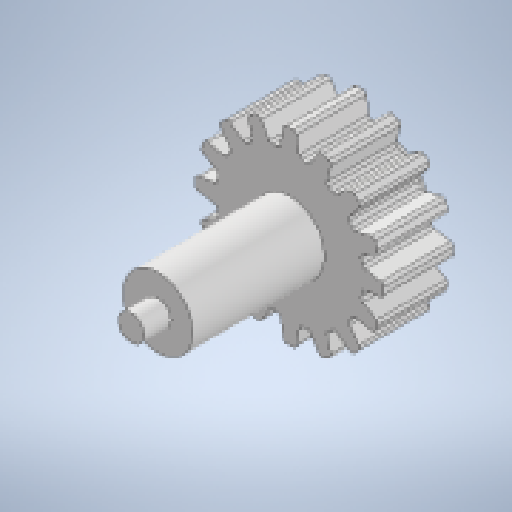
# Autodesk Inventor part: GearDirect
Saved by Autodesk Inventor 2025.2 (Build 292293000, 293)
## iProperties
Created: 2026-02-21
Part Number: GearDirect
Material: 一般
Document SubType Name: Modeling
Designer: naka6
Density: 1 g/cm^3
Appearance: 既定
Author: naka6
Autodesk Inventor part; units mm, degrees
ref_plane "YZ Plane" through (0, 0, 0) normal (1, 0, 0) x (0, 1, 0)
ref_plane "XZ Plane" through (0, 0, 0) normal (0, 1, 0) x (-1, 0, 0)
ref_plane "XY Plane" through (0, 0, 0) normal (0, 0, 1) x (1, 0, 0)
sketch "スケッチ1" plane through (0, 0, 0) normal (0, 0, 1) x (1, 0, 0)
  circle A0 centre (0, 0) radius 7 projected
  point P0 (0, 0)
extrude "押し出し1" add sketch "スケッチ1" along normal blind 3
sketch "スケッチ2" plane through (0, 0, 3) normal (0, 0, 1) x (1, 0, 0)
  circle A0 centre (0, 0) radius 13.5
  dimension "d2" = 27
  constraints: 1 centre point, 1 coincident
  measures "d2" diameter of A0
extrude "押し出し2" add sketch "スケッチ2" along normal blind 10
sketch "スケッチ3" plane through (0, 0, 13) normal (0, 0, 1) x (1, 0, 0)
  line L0 (0, 0) -> (13.5, 0)
  circle A0 centre (0, 0) radius 13.5 projected
  line L1 (0, 0) -> (13.4711, 0.8829)
  line L2 (0, 0) -> (13.3845, 1.7621)
  line L3 (0, 0) -> (13.2406, 2.6337)
  line L4 (0, 0) -> (13.04, 3.4941)
  line L5 (0, 0) -> (12.7836, 4.3394)
  line L6 (0, 0) -> (12.4724, 5.1662)
  line L7 (0, 0) -> (12.1078, 5.9709)
  line L8 (0, 0) -> (11.6913, 6.75)
  line L9 (0, 0) -> (11.2248, 7.5002)
  line L10 (0, 0) -> (10.7103, 8.2183)
  line L11 (0, 0) -> (10.1498, 8.9012)
  line L12 (0, 0) -> (9.5459, 9.5459)
  line L13 (0, 0) -> (8.9012, 10.1498)
  line L14 (0, 0) -> (8.2183, 10.7103)
  line L15 (0, 0) -> (7.5002, 11.2248)
  line L16 (0, 0) -> (6.75, 11.6913)
  line L17 (0, 0) -> (5.9709, 12.1078)
  line L18 (0, 0) -> (5.1662, 12.4724)
  line L19 (0, 0) -> (4.3394, 12.7836)
  line L20 (0, 0) -> (3.4941, 13.04)
  line L21 (0, 0) -> (2.6337, 13.2406)
  line L22 (0, 0) -> (1.7621, 13.3845)
  line L23 (0, 0) -> (0.8829, 13.4711)
  line L24 (0, 0) -> (0, 13.5)
  line L25 (0, 0) -> (-0.8829, 13.4711)
  line L26 (0, 0) -> (-1.7621, 13.3845)
  line L27 (0, 0) -> (-2.6337, 13.2406)
  line L28 (0, 0) -> (-3.4941, 13.04)
  line L29 (0, 0) -> (-4.3394, 12.7836)
  line L30 (0, 0) -> (-5.1662, 12.4724)
  line L31 (0, 0) -> (-5.9709, 12.1078)
  line L32 (0, 0) -> (-6.75, 11.6913)
  line L33 (0, 0) -> (-7.5002, 11.2248)
  line L34 (0, 0) -> (-8.2183, 10.7103)
  line L35 (0, 0) -> (-8.9012, 10.1498)
  line L36 (0, 0) -> (-9.5459, 9.5459)
  line L37 (0, 0) -> (-10.1498, 8.9012)
  line L38 (0, 0) -> (-10.7103, 8.2183)
  line L39 (0, 0) -> (-11.2248, 7.5002)
  line L40 (0, 0) -> (-11.6913, 6.75)
  line L41 (0, 0) -> (-12.1078, 5.9709)
  line L42 (0, 0) -> (-12.4724, 5.1662)
  line L43 (0, 0) -> (-12.7836, 4.3394)
  line L44 (0, 0) -> (-13.04, 3.4941)
  line L45 (0, 0) -> (-13.2406, 2.6337)
  line L46 (0, 0) -> (-13.3845, 1.7621)
  line L47 (0, 0) -> (-13.4711, 0.8829)
  line L48 (0, 0) -> (-13.5, 0)
  line L49 (0, 0) -> (-13.4711, -0.8829)
  line L50 (0, 0) -> (-13.3845, -1.7621)
  line L51 (0, 0) -> (-13.2406, -2.6337)
  line L52 (0, 0) -> (-13.04, -3.4941)
  line L53 (0, 0) -> (-12.7836, -4.3394)
  line L54 (0, 0) -> (-12.4724, -5.1662)
  line L55 (0, 0) -> (-12.1078, -5.9709)
  line L56 (0, 0) -> (-11.6913, -6.75)
  line L57 (0, 0) -> (-11.2248, -7.5002)
  line L58 (0, 0) -> (-10.7103, -8.2183)
  line L59 (0, 0) -> (-10.1498, -8.9012)
  line L60 (0, 0) -> (-9.5459, -9.5459)
  line L61 (0, 0) -> (-8.9012, -10.1498)
  line L62 (0, 0) -> (-8.2183, -10.7103)
  line L63 (0, 0) -> (-7.5002, -11.2248)
  line L64 (0, 0) -> (-6.75, -11.6913)
  line L65 (0, 0) -> (-5.9709, -12.1078)
  line L66 (0, 0) -> (-5.1662, -12.4724)
  line L67 (0, 0) -> (-4.3394, -12.7836)
  line L68 (0, 0) -> (-3.4941, -13.04)
  line L69 (0, 0) -> (-2.6337, -13.2406)
  line L70 (0, 0) -> (-1.7621, -13.3845)
  line L71 (0, 0) -> (-0.8829, -13.4711)
  line L72 (0, 0) -> (0, -13.5)
  line L73 (0, 0) -> (0.8829, -13.4711)
  line L74 (0, 0) -> (1.7621, -13.3845)
  line L75 (0, 0) -> (2.6337, -13.2406)
  line L76 (0, 0) -> (3.4941, -13.04)
  line L77 (0, 0) -> (4.3394, -12.7836)
  line L78 (0, 0) -> (5.1662, -12.4724)
  line L79 (0, 0) -> (5.9709, -12.1078)
  line L80 (0, 0) -> (6.75, -11.6913)
  line L81 (0, 0) -> (7.5002, -11.2248)
  line L82 (0, 0) -> (8.2183, -10.7103)
  line L83 (0, 0) -> (8.9012, -10.1498)
  line L84 (0, 0) -> (9.5459, -9.5459)
  line L85 (0, 0) -> (10.1498, -8.9012)
  line L86 (0, 0) -> (10.7103, -8.2183)
  line L87 (0, 0) -> (11.2248, -7.5002)
  line L88 (0, 0) -> (11.6913, -6.75)
  line L89 (0, 0) -> (12.1078, -5.9709)
  line L90 (0, 0) -> (12.4724, -5.1662)
  line L91 (0, 0) -> (12.7836, -4.3394)
  line L92 (0, 0) -> (13.04, -3.4941)
  line L93 (0, 0) -> (13.2406, -2.6337)
  line L94 (0, 0) -> (13.3845, -1.7621)
  line L95 (0, 0) -> (13.4711, -0.8829)
  circle A1 centre (0, 0) radius 10.5
  line L96 (13.4711, 0.8829) -> (10.4128, 1.3507)
  line L97 (13.4711, -0.8829) -> (10.4128, -1.3507)
  point P0 (13.4711, 0.8829)
  point P1 (13.2406, 2.6337)
  point P2 (10.2982, 2.0484)
  point P3 (13.4711, -0.8829)
  point P4 (10.2982, -2.0484)
  dimension "d7" = 360
  dimension "d9" = 21
  constraints: 196 end point, 3 coincident, 2 point on circle, 1 centre point, 1 horizontal, 289 other
  measures "d9" diameter of A1
extrude "押し出し3" cut sketch "スケッチ3" against normal through all contours A1 L3 A0 L2 | L2 A0 L96 A1 | A1 L94 A0 L93 | A1 L97 A0 L94
fillet "フィレット1" radius 0.5 4 edges at (13.4711, -0.8829, 8) (13.4711, 0.8829, 8) (10.4128, 1.3507, 8) (10.4128, -1.3507, 8)
pattern_circular "円形状パターン1" count 16 over 360 about axis through (0, 0, 3) along (0, 0, 1) of "押し出し3", "フィレット1"
sketch "スケッチ4" plane through (0, 0, 13) normal (0, 0, 1) x (1, 0, 0)
  circle A0 centre (0, 0) radius 5
  dimension "d16" = 10
  constraints: 1 centre point, 1 coincident
  measures "d16" diameter of A0
extrude "押し出し4" add sketch "スケッチ4" along normal blind 18.9
sketch "スケッチ5" plane through (0, 0, 31.9) normal (0, 0, 1) x (1, 0, 0)
  circle A0 centre (0, 0) radius 1.85
  dimension "d19" = 3.7
  constraints: 1 centre point, 1 coincident
  measures "d19" diameter of A0
extrude "押し出し5" add sketch "スケッチ5" along normal blind 3.8
